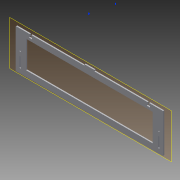
# Autodesk Inventor part: Panel_back
Saved by Autodesk Inventor 2013 (Build 170138000, 138)
## iProperties
Created: 2013-02-02
Part Number: Panel_back
Material: Aluminum 6061
Document SubType Name: Modeling
Designer: xylzlyx
Density: 1 g/cm^3
Author: xylzlyx
Autodesk Inventor part; units mm, degrees
ref_plane "YZ Plane" through (0, 0, 0) normal (1, 0, 0) x (0, 1, 0)
ref_plane "XZ Plane" through (0, 0, 0) normal (0, 1, 0) x (-1, 0, 0)
ref_plane "XY Plane" through (0, 0, 0) normal (0, 0, 1) x (1, 0, 0)
ref_plane "Work Plane1" through (-16.0071, 0, -12.7) normal (0, 0, 1) x (1, 0, 0)
sketch "Sketch1" plane through (-16.0071, 0, -12.7) normal (0, 0, 1) x (1, 0, 0)
  line L0 (0, -104.216) -> (0, -100.9921) construction
  line L1 (0, -100.9921) -> (381, -100.9921) construction
  line L2 (381, -100.9921) -> (381, -104.216) construction
  line L3 (381, -104.216) -> (0, -104.216) construction
  line L4 (381, 3.175) -> (381, 0) construction
  line L5 (381, 0) -> (0, 0) construction
  line L6 (0, 0) -> (0, 3.175) construction
  line L7 (0, 3.175) -> (381, 3.175) construction
  line L8 (381, -100.9921) -> (0, -100.9921)
  line L9 (0, -100.9921) -> (0, 0)
  line L10 (0, 0) -> (381, 0)
  line L11 (381, 0) -> (381, -100.9921)
  constraints: 24 end point, 5 horizontal, 4 coincident, 4 vertical, 2 parallel, 1 perpendicular, 7 other
extrude "BackPanel" add sketch "Sketch1" along normal blind 3.175
fillet "CornerFillet" radius 1 4 edges at (364.9929, -100.9921, -11.1125) (364.9929, 0, -11.1125) (-16.0071, 0, -11.1125) (-16.0071, -100.9921, -11.1125)
sketch "ScrewSlotSketch" plane through (-16.0071, 0, -9.525) normal (0, 0, 1) x (1, 0, 0)
  line L0 (0, -104.7759) -> (0, -101.5519) construction
  line L1 (0, -101.5519) -> (381, -101.5519) construction
  line L2 (381, -101.5519) -> (381, -104.7759) construction
  line L3 (381, -104.7759) -> (0, -104.7759) construction
  line L4 (381, 0) -> (0, 0) construction
  line L5 (0, 0) -> (0, 3.175) construction
  line L6 (0, 3.175) -> (381, 3.175) construction
  line L7 (381, 3.175) -> (381, 0) construction
  line L8 (341.0013, 3.175) -> (341.0013, -8.89)
  line L9 (341.0013, 3.175) -> (344.7986, 3.175)
  line L10 (344.7986, 3.175) -> (344.7986, -8.89)
  line L11 (344.7986, -8.89) -> (341.0013, -8.89)
  line L12 (342.9, -8.89) -> (342.9, 3.175) construction
  line L13 (346.9957, -8.89) -> (338.8042, -8.89)
  line L14 (338.8042, -8.89) -> (338.8042, -5.8579)
  line L15 (338.8042, -5.8579) -> (346.9957, -5.8579)
  line L16 (346.9957, -5.8579) -> (346.9957, -8.89)
  line L17 (36.2014, -8.89) -> (36.2014, 3.175)
  line L18 (36.2014, 3.175) -> (39.9987, 3.175)
  line L19 (39.9987, 3.175) -> (39.9987, -8.89)
  line L20 (39.9987, -8.89) -> (36.2014, -8.89)
  line L21 (42.1958, -8.89) -> (34.0043, -8.89)
  line L22 (42.1958, -8.89) -> (42.1958, -5.8579)
  line L23 (42.1958, -5.8579) -> (34.0043, -5.8579)
  line L24 (34.0043, -5.8579) -> (34.0043, -8.89)
  line L25 (368.3, -48.0974) -> (368.3, -1) projected
  line L26 (12.7, -1) -> (12.7, -48.0974) projected
  line L27 (368.3, -48.0974) -> (368.3, -1) projected
  point P0 (16.0071, 0)
  point P1 (38.1, 3.175)
  point P2 (38.1, -8.89)
  dimension "d3" = 12.065
  dimension "d5" = 3.7973
  dimension "d7" = 8.1915
  dimension "d8" = 3.0321
  dimension "d9" = 12.065
  dimension "d10" = 3.7973
  dimension "d12" = 8.1915
  dimension "d13" = 3.0321
  dimension "d22" = 25.4
  dimension "d23" = 25.4
  constraints: 50 end point, 13 parallel, 6 midpoint, 4 horizontal, 4 vertical, 3 collinear, 2 point on line, 1 perpendicular, 8 other
  measures "d3" distance of L8.start L8.end
  measures "d5" distance of L8.start L9.end
  measures "d7" distance of L13.start L13.end
  measures "d8" distance of L15.end L13.start
  measures "d9" distance of L17.start L17.end
  measures "d10" distance of L17.end L18.end
  measures "d12" distance of L21.start L21.end
  measures "d13" distance of L21.start L22.end
  measures "d22" distance between parallel lines of L12 L25
  measures "d23" distance from line of L26 point (38.1, 3.175)
extrude "ScrewSlotExtrusion" cut sketch "ScrewSlotSketch" against normal blind 3.175
fillet "SlotFillets" radius 0.5 16 edges at (328.7916, -5.8579, -11.1125) (328.7916, 0, -11.1125) (324.9943, 0, -11.1125) (324.9943, -5.8579, -11.1125) (330.9887, -5.8579, -11.1125) (322.7972, -5.8579, -11.1125) (330.9887, -8.89, -11.1125) (322.7972, -8.89, -11.1125) (20.1943, -5.8579, -11.1125) (17.9972, -5.8579, -11.1125) (20.1943, 0, -11.1125) (17.9972, -8.89, -11.1125) (23.9916, -5.8579, -11.1125) (23.9916, 0, -11.1125) (26.1887, -8.89, -11.1125) (26.1887, -5.8579, -11.1125)
sketch "ScrewHoleSketch" plane through (-16.0071, 0, -9.525) normal (0, 0, 1) x (1, 0, 0)
  line L0 (188.6013, -6.4929) -> (188.6013, 0) projected
  line L1 (368.3, -48.5974) -> (371.475, -48.5974) projected
  line L2 (371.475, -52.3947) -> (368.3, -52.3947) projected
  line L3 (12.7, -52.3947) -> (9.525, -52.3947) projected
  line L4 (9.525, -48.5974) -> (12.7, -48.5974) projected
  line L5 (368.3, -48.5974) -> (368.3, -52.3947) construction
  line L6 (12.7, -48.5974) -> (12.7, -52.3947) construction
  point P0 (188.6013, -5.9929)
  point P1 (188.6013, -0.5)
  point P2 (16.0071, 0)
  point P3 (369.8875, -50.496)
  point P4 (11.1125, -50.496)
  point P5 (368.3, -50.496)
  point P6 (369.8875, -48.5974)
  point P7 (11.1125, -48.5974)
  point P8 (12.7, -50.496)
  constraints: 4 end point, 4 midpoint, 2 horizontal alignment, 2 parallel, 2 vertical alignment
hole "Hole1" at (353.8804, -50.496, -9.525) at (-4.8946, -50.496, -9.525) direction (0, 0, -1) diameter 3.7973 end through all
sketch "BottomTabSketch" plane through (24.4916, 0, -12.7) normal (0, 1, 0) x (1, 0, 0)
  line L0 (137.3013, -3.175) -> (162.7013, -3.175)
  line L1 (162.7013, -3.175) -> (162.7013, 0)
  line L2 (162.7013, 0) -> (137.3013, 0)
  line L3 (137.3013, 0) -> (137.3013, -3.175)
  line L4 (136.6663, -0.1825) -> (136.6663, -2.9925) projected
  line L5 (137.1663, -3.4925) -> (162.8363, -3.4925) projected
  point P0 (0, 0)
  point P1 (-24.4916, -12.7)
  point P2 (150.0013, -3.4925)
  point P3 (150.0013, -3.175)
  point P4 (137.3013, -1.5875)
  point P5 (136.6663, -1.5875)
  dimension "d32" = 25.4
  constraints: 8 end point, 4 midpoint, 2 horizontal alignment, 2 parallel, 1 horizontal, 1 perpendicular, 1 vertical alignment
  measures "d32" distance of L1.end L2.end
extrude "BottomTab" add sketch "BottomTabSketch" along normal blind 3.175
fillet "BottomTabFillet" radius 0.5 4 edges at (161.7929, 0, -11.1125) (161.7929, 3.175, -11.1125) (187.1929, 0, -11.1125) (187.1929, 3.175, -11.1125)
sketch "SlotSketch" plane through (-16.0071, 0, -9.525) normal (0, 0, 1) x (1, 0, 0)
  circle A0 centre (369.8875, -50.496) radius 1.8986 projected
  circle A1 centre (11.1125, -50.496) radius 1.8986 projected
  line L0 (0, -104.7759) -> (0, -101.5519) construction
  line L1 (0, -101.5519) -> (381, -101.5519) construction
  line L2 (381, -101.5519) -> (381, -104.7759) construction
  line L3 (381, -104.7759) -> (0, -104.7759) construction
  line L4 (371.7925, -89.0791) -> (367.9825, -89.0791)
  line L5 (367.9825, -89.0791) -> (367.9825, -62.4091)
  line L6 (367.9825, -62.4091) -> (371.7925, -62.4091)
  line L7 (371.7925, -62.4091) -> (371.7925, -89.0791)
  line L8 (13.0175, -89.0791) -> (9.2075, -89.0791)
  line L9 (9.2075, -89.0791) -> (9.2075, -62.4091)
  line L10 (9.2075, -62.4091) -> (13.0175, -62.4091)
  line L11 (13.0175, -62.4091) -> (13.0175, -89.0791)
  line L12 (1, -100.9921) -> (380, -100.9921) projected
  line L13 (203.2, 0.5) -> (203.2, 2.675) projected
  line L14 (11.1125, -50.496) -> (11.1125, -100.9921) construction
  line L15 (369.8875, -50.496) -> (369.8875, -100.9921) construction
  point P0 (16.0071, 0)
  point P1 (11.1125, -75.7441)
  point P2 (13.0175, -75.7441)
  point P3 (11.1125, -62.4091)
  point P4 (369.8875, -75.7441)
  point P5 (371.7925, -75.7441)
  point P6 (369.8875, -62.4091)
  dimension "d37" = 26.67
  dimension "d39" = 3.81
  dimension "d40" = 26.67
  dimension "d41" = 3.81
  constraints: 28 end point, 6 midpoint, 6 parallel, 4 horizontal, 2 horizontal alignment, 2 perpendicular, 2 point on line, 2 vertical, 2 vertical alignment, 4 other
  measures "d37" distance of L4.end L5.end
  measures "d39" distance of L4.start L4.end
  measures "d40" distance of L10.end L8.start
  measures "d41" distance of L8.start L8.end
extrude "Slots" cut sketch "SlotSketch" against normal blind 3.175 contours L4 L5 L6 L7 | L8 L9 L10 L11
fillet "Fillet4" radius 0.5 8 edges at (355.7854, -89.0791, -11.1125) (351.9754, -89.0791, -11.1125) (351.9754, -62.4091, -11.1125) (355.7854, -62.4091, -11.1125) (-6.7996, -62.4091, -11.1125) (-2.9896, -62.4091, -11.1125) (-6.7996, -89.0791, -11.1125) (-2.9896, -89.0791, -11.1125)
sketch "Sketch6" plane through (-16.0071, 0, -9.525) normal (0, 0, 1) x (1, 0, 0)
  line L0 (1, -100.9921) -> (380, -100.9921) projected
  line L1 (380, 0) -> (345.2986, 0) projected
  circle A0 centre (369.8875, -50.496) radius 1.8986 projected
  circle A1 centre (11.1125, -50.496) radius 1.8986 projected
  line L2 (354.6475, -85.7521) -> (26.3525, -85.7521)
  line L3 (26.3525, -85.7521) -> (26.3525, -15.24)
  line L4 (26.3525, -15.24) -> (354.6475, -15.24)
  line L5 (354.6475, -15.24) -> (354.6475, -85.7521)
  point P0 (16.0071, 0)
  dimension "d45" = 15.24
  dimension "d46" = 15.24
  dimension "d47" = 15.24
  dimension "d48" = 15.24
  constraints: 8 end point, 2 parallel, 1 horizontal, 1 perpendicular
  measures "d45" distance from line of L0 L2.start
  measures "d46" distance from line of L1 L4.end
  measures "d47" distance from line of A0.centre L5
  measures "d48" horizontal distance of A1.centre L3.end
extrude "InsideGap" cut sketch "Sketch6" against normal blind 25.4 contours L2 L3 L4 L5
fillet "InsideGapFillet" radius 0.5 4 edges at (338.6404, -85.7521, -11.1125) (338.6404, -15.24, -11.1125) (10.3454, -15.24, -11.1125) (10.3454, -85.7521, -11.1125)
equation "\"d3\" = ScrewLen"
equation "\"d5\" = ScrewHoleD"
equation "\"d7\" = NutFlatsGap"
equation "\"d8\" = NutHeightGap"
equation "\"d9\" = ScrewLen"
equation "\"d10\" = ScrewHoleD"
equation "\"d12\" = NutFlatsGap"
equation "\"d13\" = NutHeightGap"
equation "\"d22\" = ScrewHoleDist"
equation "\"d23\" = ScrewHoleDist"
equation "\"d24\" = SlotFilletRad"
equation "\"d25\" = ScrewHoleD"
equation "\"d32\" = TabLength"
equation "\"d36\" = SlotFilletRad"
equation "\"d37\" = SlotLength"
equation "\"d39\" = SlotWidth"
equation "\"d40\" = SlotLength"
equation "\"d41\" = SlotWidth"
equation "\"d44\" = SlotFilletRad"
equation "\"d45\" = EdgeThickness"
equation "\"d46\" = EdgeThickness"
equation "\"d47\" = EdgeThickness"
equation "\"d48\" = EdgeThickness"
equation "\"d51\" = SlotFilletRad"
equation "\"ScrewLen\" = 12.065"
equation "\"ScrewHoleD\" = 3.7973"
equation "\"NutFlatsGap\" = 8.1915"
equation "\"NutHeightGap\" = 3.032125"
equation "\"ScrewHoleDist\" = 25.4"
equation "\"SlotFilletRad\" = 0.5"
equation "\"TabLength\" = 25.4"
equation "\"SlotLength\" = 26.67"
equation "\"SlotWidth\" = 3.81"
equation "\"EdgeThickness\" = 15.24"
body "Solid1"
